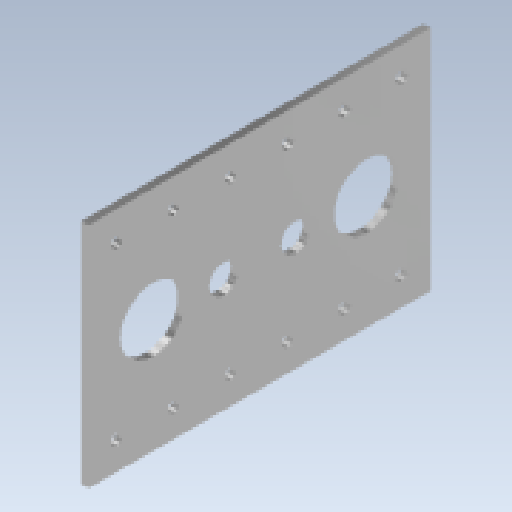
# Autodesk Inventor part: CH-1-02-RearGearboxHousingMotorSide
Saved by Autodesk Inventor 2023 (Build 270158000, 158)
## iProperties
Created: 2023-02-05
Part Number: CH-1-02-RearGearboxHousingMotorSide
Material: Aluminum 6061
Document SubType Name: Modeling
Designer: Dave
Density: 2.7 g/cm^3
Appearance: Chrome - Polished
Mass: 117.299 g
Surface Area: 304.37 cm^2
Volume: 43.444 cm^3
Author: Dave
Autodesk Inventor part; units mm, degrees
ref_plane "YZ Plane" through (0, 0, 0) normal (1, 0, 0) x (0, 1, 0)
ref_plane "XZ Plane" through (0, 0, 0) normal (0, 1, 0) x (-1, 0, 0)
ref_plane "XY Plane" through (0, 0, 0) normal (0, 0, 1) x (1, 0, 0)
sketch "Sketch1" plane through (0, 0, 0) normal (1, 0, 0) x (0, 1, 0)
  line L0 (0, 0) -> (101.6, 0)
  line L1 (101.6, 0) -> (101.6, -152.4)
  line L2 (101.6, -152.4) -> (0, -152.4)
  line L3 (0, -152.4) -> (0, 0)
  circle A0 centre (50.8, -28.575) radius 14.2875
  circle A1 centre (50.8, -60.325) radius 6.35
  circle A2 centre (50.8, -92.075) radius 6.35
  circle A3 centre (50.8, -123.825) radius 14.2875
  line L4 (50.8, -28.575) -> (50.8, -123.825) construction
  circle A4 centre (88.9, -12.7) radius 2.65
  circle A5 centre (88.9, -38.1) radius 2.65
  circle A6 centre (88.9, -63.5) radius 2.65
  circle A7 centre (88.9, -88.9) radius 2.65
  circle A8 centre (88.9, -114.3) radius 2.65
  circle A9 centre (88.9, -139.7) radius 2.65
  circle A10 centre (12.7, -12.7) radius 2.65
  circle A11 centre (12.7, -38.1) radius 2.65
  circle A12 centre (12.7, -63.5) radius 2.65
  circle A13 centre (12.7, -88.9) radius 2.65
  circle A14 centre (12.7, -114.3) radius 2.65
  circle A15 centre (12.7, -139.7) radius 2.65
  point P0 (101.6, -76.2)
  point P1 (50.8, -76.2)
  point P2 (50.8, -152.4)
  dimension "d0" = 101.6
  dimension "d1" = 152.4
  dimension "d2" = 28.575
  dimension "d3" = 12.7
  dimension "d4" = 12.7
  dimension "d5" = 28.575
  dimension "d6" = 31.75
  dimension "d7" = 31.75
  dimension "d8" = 31.75
  dimension "d9" = 5.3
  dimension "d10" = 12.7
  dimension "d11" = 12.7
  dimension "d14" = 25.4
  dimension "d17" = 76.2
  constraints: 16 centre point, 10 end point, 4 vertical alignment, 3 midpoint, 2 horizontal, 2 parallel, 2 vertical, 1 horizontal alignment, 1 perpendicular, 22 other
  measures "d0" distance of L1.end L2.end
  measures "d1" distance of L0.end L1.end
  measures "d2" diameter of A0
  measures "d3" diameter of A1
  measures "d4" diameter of A2
  measures "d5" diameter of A3
  measures "d6" distance of A1.centre L4.start
  measures "d7" distance of A2.centre A1.centre
  measures "d8" distance of A2.centre L4.end
  measures "d9" diameter of A4
  measures "d10" distance from line of L1 A4.centre
  measures "d11" distance from line of L0 A4.centre
  measures "d14" distance of A4.centre A5.centre
  measures "d17" distance of A4.centre A10.centre
extrude "Extrusion1" add sketch "Sketch1" along normal blind 3.175
equation "\"d7\" = d6"
equation "\"d8\" = d7"
body "Solid1"
